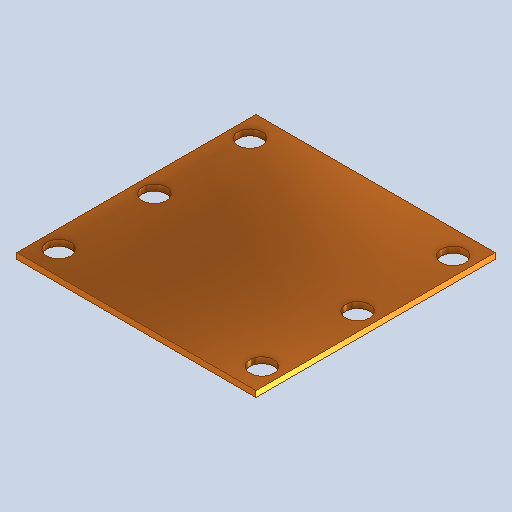
# Autodesk Inventor part: 26A
Saved by Autodesk Inventor 2025.1 (Build 291241000, 241)
## iProperties
Created: 2024-09-17
Part Number: 26A
Material: Gold
Document SubType Name: Modeling
Designer: ffogue
Density: 19.3 g/cm^3
Appearance: Metal 1600F Hot
Author: ffogue
Autodesk Inventor part; units mm, degrees
ref_plane "YZ Plane" through (0, 0, 0) normal (1, 0, 0) x (0, 1, 0)
ref_plane "XZ Plane" through (0, 0, 0) normal (0, 1, 0) x (-1, 0, 0)
ref_plane "XY Plane" through (0, 0, 0) normal (0, 0, 1) x (1, 0, 0)
sketch "Sketch1" plane through (0, 0, 0) normal (0, 0, 1) x (1, 0, 0)
  line L0 (-20, -20) -> (20, -20)
  line L1 (20, -20) -> (20, 20)
  line L2 (20, 20) -> (-20, 20)
  line L3 (-20, 20) -> (-20, -20)
  line L4 (-20, -20) -> (20, 20) construction
  line L5 (20, -20) -> (-20, 20) construction
  point P0 (0, 0)
  dimension "d0" = 40
  dimension "d1" = 40
  constraints: 12 end point, 2 midpoint, 2 parallel, 1 horizontal, 1 perpendicular
  measures "d0" distance of L1.end L2.end
  measures "d1" distance of L2.end L0.start
extrude "Extrusion1" add sketch "Sketch1" along normal mid plane 1
sketch "Sketch2" plane through (0, 0, 0.5) normal (0, 0, 1) x (1, 0, 0)
  circle A0 centre (-17, 16) radius 2
  circle A1 centre (-17, 0) radius 2
  circle A2 centre (-17, -16) radius 2
  circle A3 centre (17, 16) radius 2
  circle A4 centre (17, 0) radius 2
  circle A5 centre (17, -16) radius 2
  line L0 (-20, 20) -> (-20, -20) projected
  point P0 (0, 0)
  dimension "d4" = 3
  dimension "d5" = 34
  dimension "d6" = 4
  dimension "d7" = 4
  dimension "d8" = 4
  dimension "d9" = 16
  dimension "d10" = 32
  constraints: 6 centre point, 4 horizontal alignment, 4 vertical alignment, 3 equal radius
  measures "d4" distance from line of L0 A0.centre
  measures "d5" distance of A3.centre A0.centre
  measures "d6" diameter of A0
  measures "d7" diameter of A1
  measures "d8" diameter of A2
  measures "d9" distance of A1.centre A0.centre
  measures "d10" distance of A2.centre A0.centre
extrude "Extrusion2" cut sketch "Sketch2" against normal up to surface (1 mm away)
equation "\"d7\" = d6"
equation "\"d8\" = d6"
equation "\"d9\" = 0.5 * d10"
body "Solid1"
